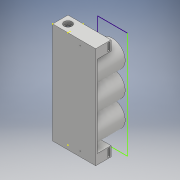
# Autodesk Inventor part: rearAxelHolder 11-28
Saved by Autodesk Inventor 2018 (Build 220112000, 112)
## iProperties
Created: 2019-11-28
Part Number: rearAxelHolder 11-28
Material: Generic
Document SubType Name: Modeling
Designer: Aditya Kendre
Density: 1 g/cm^3
Appearance: Default
Author: Aditya Kendre
Autodesk Inventor part; units mm, degrees
ref_plane "YZ Plane" through (0, 0, 0) normal (1, 0, 0) x (0, 1, 0)
ref_plane "XZ Plane" through (0, 0, 0) normal (0, 1, 0) x (-1, 0, 0)
ref_plane "XY Plane" through (0, 0, 0) normal (0, 0, 1) x (1, 0, 0)
sketch "Sketch1" plane through (0, 0, 0) normal (0, 1, 0) x (-1, 0, 0)
  line L0 (0, 0) -> (25, 0)
  line L1 (25, 0) -> (25, -165)
  line L2 (25, -165) -> (0, -165)
  line L3 (0, -165) -> (0, 0)
  dimension "d0" = 25
  dimension "d1" = 165
  constraints: 8 end point, 2 parallel, 1 horizontal, 1 perpendicular
  measures "d0" distance of L1.end L2.end
  measures "d1" distance of L0.end L1.end
extrude "Extrusion1" add sketch "Sketch1" along normal blind 3
sketch "Sketch2" plane through (0, 3, 0) normal (0, 1, 0) x (1, 0, 0)
  line L0 (-25, 165) -> (-25, 0) projected
  line L1 (0, 0) -> (0, 165) projected
  line L2 (-25, 0) -> (0, 0)
  line L3 (0, 0) -> (0, 7)
  line L4 (0, 7) -> (-25, 7)
  line L5 (-25, 7) -> (-25, 0)
  line L6 (0, 165) -> (-25, 165) projected
  line L7 (-25, 165) -> (0, 165)
  line L8 (0, 165) -> (0, 158)
  line L9 (0, 158) -> (-25, 158)
  line L10 (-25, 158) -> (-25, 165)
  dimension "d4" = 7
  dimension "d5" = 7
  constraints: 16 end point, 4 parallel, 2 horizontal, 2 perpendicular, 2 point on line
  measures "d4" distance of L3.end L2.end
  measures "d5" distance of L7.end L8.end
extrude "Extrusion2" add sketch "Sketch2" along normal blind 22 contours L6 L1 L9 L0 | L4 L1 L2 L0
sketch "Sketch3" plane through (-25, 0, 0) normal (0, 0, 1) x (1, 0, 0)
  point P0 (25, 0)
sketch "Sketch4" plane through (-25, 0, 0) normal (0, 0, 1) x (1, 0, 0)
  line L0 (25, 25) -> (0, 25) construction
  line L1 (25, 0) -> (0, 25) construction
  circle A0 centre (12.5, 12.5) radius 6.5
  dimension "d8" = 13
  constraints: 2 end point, 1 centre point, 1 coincident, 1 midpoint
  measures "d8" diameter of A0
extrude "Extrusion3" cut sketch "Sketch4" against normal blind 5
sketch "Sketch5" plane through (0, 0, -165) normal (0, 0, -1) x (-1, 0, 0)
  circle A0 centre (12.5, 12.5) radius 6.5 projected
  circle A1 centre (12.5, 12.5) radius 6.5
  point P0 (0, 0)
  constraints: 1 centre point, 1 coincident
extrude "Extrusion4" cut sketch "Sketch5" against normal blind 5
sketch "Sketch6" plane through (-25, 0, 0) normal (0, 0, 1) x (1, 0, 0)
  circle A0 centre (12.5, 12.5) radius 6.5 projected
  circle A1 centre (12.5, 12.5) radius 5
  point P0 (25, 0)
  dimension "d13" = 10
  constraints: 1 centre point, 1 coincident
  measures "d13" diameter of A1
extrude "Extrusion5" cut sketch "Sketch6" against normal blind 165 contours A1
sketch "Sketch7" plane through (-25, 3, -158) normal (0, 0, 1) x (1, 0, 0)
  line L0 (25, 0) -> (25, 22) construction
  line L1 (0, 0) -> (0, 22) construction
  point P0 (25, -3)
sketch "Sketch8" plane through (-25, 3, -158) normal (0, 0, 1) x (1, 0, 0)
  circle A0 centre (12.5, 9.5) radius 5 projected
  point P0 (25, -3)
  constraints: 1 coincident
sketch "Sketch9" plane through (0, 3, 0) normal (0, 1, 0) x (1, 0, 0)
  line L0 (-25, 158) -> (0, 158) projected
  line L1 (0, 7) -> (-25, 7) projected
  line L2 (-25, 158) -> (-20, 158)
  line L3 (-20, 158) -> (-20, 7)
  line L4 (-20, 7) -> (-25, 7)
  line L5 (-25, 7) -> (-25, 158)
  line L6 (0, 0) -> (0, 7) projected
  line L7 (0, 7) -> (-5, 7)
  line L8 (-5, 7) -> (-5, 158)
  line L9 (-5, 158) -> (0, 158)
  line L10 (0, 158) -> (0, 7)
  dimension "d16" = 5
  dimension "d17" = 5
  constraints: 16 end point, 4 parallel, 2 horizontal, 2 perpendicular, 2 point on line
  measures "d16" distance of L3.end L4.end
  measures "d17" distance of L8.end L9.end
extrude "Extrusion6" add sketch "Sketch9" along normal blind 7.5 contours L0 L3 L1 L5 | L0 L10 L1 L8
fillet "Fillet1" radius 2 2 edges at (-5, 10.5, -82.5) (-20, 10.5, -82.5)
sketch "Sketch10" plane through (0, 0, 0) normal (1, 0, 0) x (0, 0, -1)
  line L0 (165, 0) -> (165, 25) projected
  line L1 (0, 0) -> (165, 0)
  line L2 (165, 0) -> (165, 3)
  line L3 (165, 3) -> (0, 3)
  line L4 (0, 3) -> (0, 0)
  dimension "d21" = 3
  constraints: 8 end point, 2 parallel, 1 horizontal, 1 perpendicular, 1 point on line
  measures "d21" distance of L2.end L1.end
extrude "Extrusion7" add sketch "Sketch10" along normal blind 45
sketch "Sketch11" plane through (0, 3, 0) normal (0, 1, 0) x (1, 0, 0)
  line L0 (45, 165) -> (45, 0) construction
  line L1 (0, 165) -> (-25, 165) construction
  line L2 (45, 82.5) -> (3, 82.5) construction
  circle A0 centre (24, 82.5) radius 21 construction
  circle A1 centre (24, 124.5) radius 21 construction
  circle A2 centre (24, 124.5) radius 21
  circle A3 centre (24, 82.5) radius 21
  circle A4 centre (24, 40.5) radius 21
  circle A5 centre (24, 40.5) radius 19.325
  circle A6 centre (24, 82.5) radius 19.325
  circle A7 centre (24, 124.5) radius 19.325
  point P0 (0, 0)
  dimension "d24" = 42
  dimension "d25" = 38.65
  dimension "d26" = 38.65
  dimension "d27" = 38.65
  constraints: 7 centre point, 5 coincident, 2 end point, 2 midpoint, 1 concentric, 1 equal radius, 1 horizontal, 1 horizontal alignment, 4 other
  measures "d24" distance of L2.start L2.end
  measures "d25" diameter of A5
  measures "d26" diameter of A6
  measures "d27" diameter of A7
extrude "Extrusion8" add sketch "Sketch11" along normal blind 45
sketch "Sketch12" plane through (0, 3, 0) normal (0, 1, 0) x (1, 0, 0)
  point P0 (0, 0)
sketch "Sketch13" plane through (0, 3, 0) normal (0, 1, 0) x (1, 0, 0)
  line L0 (45, 40.5) -> (45, 0) projected
  line L1 (0, 0) -> (0, 165) projected
  line L2 (45, 0) -> (0, 0)
  line L3 (0, 0) -> (0, 16)
  line L4 (0, 16) -> (45, 16)
  line L5 (45, 16) -> (45, 0)
  line L6 (45, 165) -> (45, 124.5) projected
  line L7 (0, 165) -> (45, 165)
  line L8 (45, 165) -> (45, 149)
  line L9 (45, 149) -> (0, 149)
  line L10 (0, 149) -> (0, 165)
  dimension "d30" = 16
  dimension "d31" = 16
  constraints: 16 end point, 4 parallel, 2 horizontal, 2 perpendicular, 2 point on line
  measures "d30" distance of L2.end L3.end
  measures "d31" distance of L7.end L8.end
extrude "Extrusion9" add sketch "Sketch13" along normal blind 22
sketch "Sketch14" plane through (45, 0, 0) normal (1, 0, 0) x (0, 0, -1)
  line L0 (0, 25) -> (16, 25) construction
  line L1 (8, 25) -> (8, 21.5) construction
  line L2 (14.125, 23.125) -> (1.875, 23.125)
  line L3 (1.875, 23.125) -> (1.875, 19.875)
  line L4 (1.875, 19.875) -> (14.125, 19.875)
  line L5 (14.125, 19.875) -> (14.125, 23.125)
  line L6 (14.125, 23.125) -> (1.875, 19.875) construction
  line L7 (1.875, 23.125) -> (14.125, 19.875) construction
  point P0 (0, 0)
  dimension "d35" = 3.5
  dimension "d36" = 12.25
  dimension "d37" = 3.25
  constraints: 14 end point, 3 midpoint, 2 parallel, 1 horizontal, 1 perpendicular, 1 vertical
  measures "d35" distance of L1.start L1.end
  measures "d36" distance of L4.end L3.end
  measures "d37" distance of L3.end L2.end
sketch "Sketch15" plane through (45, 0, 0) normal (1, 0, 0) x (0, 0, -1)
  line L0 (149, 25) -> (165, 25) construction
  line L1 (157, 25) -> (157, 21.5) construction
  line L2 (163.125, 23.125) -> (150.875, 23.125)
  line L3 (150.875, 23.125) -> (150.875, 19.875)
  line L4 (150.875, 19.875) -> (163.125, 19.875)
  line L5 (163.125, 19.875) -> (163.125, 23.125)
  line L6 (163.125, 23.125) -> (150.875, 19.875) construction
  line L7 (150.875, 23.125) -> (163.125, 19.875) construction
  point P0 (0, 0)
  dimension "d38" = 3.5
  dimension "d39" = 12.25
  dimension "d40" = 3.25
  constraints: 14 end point, 3 midpoint, 2 parallel, 1 horizontal, 1 perpendicular, 1 vertical
  measures "d38" distance of L1.start L1.end
  measures "d39" distance of L4.end L3.end
  measures "d40" distance of L3.end L2.end
extrude "Extrusion10" cut sketch "Sketch14" against normal blind 40
extrude "Extrusion11" cut sketch "Sketch15" against normal blind 40
sketch "Sketch16" plane through (0, 25, 0) normal (0, 1, 0) x (1, 0, 0)
  line L0 (45, 0) -> (45, 16) construction
  line L1 (45, 8) -> (20, 8) construction
  circle A0 centre (20, 8) radius 0.75 construction
  circle A1 centre (20, 8) radius 0.75
  point P0 (0, 0)
  dimension "d45" = 25
  dimension "d46" = 1.5
  constraints: 2 centre point, 2 coincident, 2 end point, 1 horizontal, 1 midpoint
  measures "d45" distance of L1.start L1.end
  measures "d46" diameter of A0
extrude "Extrusion12" cut sketch "Sketch16" against normal blind 25
sketch "Sketch17" plane through (0, 25, 0) normal (0, 1, 0) x (1, 0, 0)
  point P0 (0, 0)
sketch "Sketch18" plane through (0, 25, 0) normal (0, 1, 0) x (1, 0, 0)
  point P0 (0, 0)
sketch "Sketch19" plane through (0, 25, 0) normal (0, 1, 0) x (1, 0, 0)
  point P0 (0, 0)
sketch "Sketch20" plane through (0, 25, 0) normal (0, 1, 0) x (1, 0, 0)
  line L0 (0, 149) -> (45, 149) construction
  line L1 (45, 0) -> (45, 165) construction
  line L2 (45, 149) -> (45, 165) construction
  line L3 (45, 157) -> (20, 157) construction
  circle A0 centre (20, 157) radius 0.75
  point P0 (0, 0)
  dimension "d49" = 25
  dimension "d50" = 1.5
  constraints: 4 end point, 1 centre point, 1 coincident, 1 collinear, 1 horizontal, 1 midpoint
  measures "d49" distance of L3.start L3.end
  measures "d50" diameter of A0
extrude "Extrusion13" cut sketch "Sketch20" against normal blind 25
sketch "Sketch21" plane through (-25, 0, -165) normal (-1, 0, 0) x (0, 0, 1)
  point P0 (165, 0)
sketch "Sketch22" plane through (-25, 0, -165) normal (-1, 0, 0) x (0, 0, 1)
  line L0 (158, 8.5) -> (7, 8.5) construction
  line L1 (82.5, 8.5) -> (82.5, 6.5) construction
  circle A0 centre (82.5, 6.5) radius 0.5
  point P0 (165, 0)
  dimension "d53" = 2
  dimension "d54" = 1
  constraints: 2 end point, 1 centre point, 1 coincident, 1 midpoint, 1 vertical
  measures "d53" distance of L1.start L1.end
  measures "d54" diameter of A0
extrude "Extrusion14" cut sketch "Sketch22" against normal blind 5.25
fillet "Fillet2" radius 1 1 edges at (-25, 6.5, -83)
sketch "Sketch23" plane through (-25, 0, -165) normal (-1, 0, 0) x (0, 0, 1)
  circle A0 centre (82.5, 9.5843) radius 0.5
  point P0 (165, 0)
  dimension "d58" = 1
  constraints: 1 centre point
  measures "d58" diameter of A0
extrude "Extrusion15" cut sketch "Sketch23" against normal blind 5.25
sketch "Sketch24" plane through (0, 48, 0) normal (0, 1, 0) x (1, 0, 0)
  line L0 (0, 0) -> (48.5926, 0)
  line L1 (48.5926, 0) -> (48.5926, 173.5031)
  line L2 (48.5926, 173.5031) -> (0, 173.5031)
  line L3 (0, 173.5031) -> (0, 0)
  constraints: 8 end point, 2 parallel, 1 horizontal, 1 perpendicular
body "Solid1"
